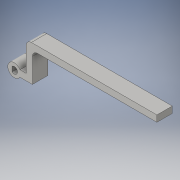
# Autodesk Inventor part: Rotator
Saved by Autodesk Inventor 2016 SP1 (Build 200210100, 210)
## iProperties
Created: 2016-04-06
Part Number: Rotator
Material: Generic
Document SubType Name: Modeling
Designer: jmehta38
Density: 1 g/cm^3
Appearance: Default
Author: jmehta38
Autodesk Inventor part; units mm, degrees
ref_plane "YZ Plane" through (0, 0, 0) normal (1, 0, 0) x (0, 1, 0)
ref_plane "XZ Plane" through (0, 0, 0) normal (0, 1, 0) x (-1, 0, 0)
ref_plane "XY Plane" through (0, 0, 0) normal (0, 0, 1) x (1, 0, 0)
sketch "Sketch2" plane through (0, 0, 0) normal (0, 0, 1) x (1, 0, 0)
  circle A0 centre (0, 0) radius 2
  circle A1 centre (0, 0) radius 4
  line L0 (3.4641, 2) -> (6.0041, 2)
  line L1 (6.0041, 2) -> (6.0041, -2.0132)
  line L2 (6.0041, -2.0132) -> (3.4564, -2.0132)
  line L3 (-1.3208, -1.5018) -> (-1.3208, 1.5018)
  dimension "d7" = 4
  dimension "d8" = 8
  dimension "d9" = 2.54
  dimension "d10" = 4.0132
  dimension "d11" = 2
  dimension "d25" = 1.3208
  constraints: 8 end point, 4 point on circle, 2 centre point, 2 coincident, 2 perpendicular, 1 horizontal, 1 vertical
  measures "d7" diameter of A0
  measures "d8" diameter of A1
  measures "d9" distance of L0.start L0.end
  measures "d10" distance of L0.end L1.end
  measures "d11" distance from line of L0 A0.centre
  measures "d25" distance from line of L3 point (0, 0)
extrude "Extrusion2" add sketch "Sketch2" along normal blind 9.398
sketch "Sketch3" plane through (6.0041, -2.0132, 0) normal (1, 0, 0) x (0, 0, -1)
  line L0 (-9.398, 0) -> (-9.398, 4.0132) projected
  line L1 (-9.398, 4.0132) -> (-9.398, 0)
  line L2 (-9.398, 0) -> (0, 0)
  line L3 (0, 0) -> (0, 4.0132) projected
  line L4 (0, 0) -> (0, 4.0132)
  line L5 (0, 4.0132) -> (-9.398, 4.0132) projected
  line L6 (0, 4.0132) -> (-9.398, 4.0132)
  point P0 (0, 2.0132)
  constraints: 8 end point, 3 perpendicular, 1 collinear
extrude "Extrusion3" add sketch "Sketch3" along normal blind 5.08
sketch "Sketch4" plane through (3.4641, 2, 9.398) normal (0, 1, 0) x (1, 0, 0)
  line L0 (0, 0) -> (7.62, 0) projected
  line L1 (7.62, 0) -> (3.81, 0)
  line L2 (3.81, 0) -> (3.81, 9.398)
  line L3 (3.81, 9.398) -> (7.62, 9.398)
  line L4 (7.62, 9.398) -> (7.62, 0)
  point P0 (-3.4641, 9.398)
  dimension "d16" = 3.81
  dimension "d17" = 9.398
  constraints: 8 end point, 3 perpendicular, 1 midpoint
  measures "d16" distance of L0.end L1.end
  measures "d17" distance between parallel lines of L3 L0
extrude "Extrusion4" add sketch "Sketch4" along normal blind 17.9303
sketch "Sketch5" plane through (11.0841, -2.0132, 0) normal (1, 0, 0) x (0, 0, -1)
  line L0 (0, 21.9435) -> (0, 18.04)
  line L1 (0, 18.04) -> (-9.398, 18.04)
  line L2 (-9.398, 18.04) -> (-9.398, 21.9435)
  line L3 (0, 0) -> (0, 21.9435) projected
  line L4 (-9.398, 21.9435) -> (0, 21.9435)
  point P0 (0, 2.0132)
  point P1 (-9.398, 21.9435)
  dimension "d29" = 9.398
  dimension "d30" = 3.9035
  dimension "d31" = 3.9035
  constraints: 8 end point, 2 perpendicular, 1 vertical
  measures "d29" distance of L0.end L1.end
  measures "d30" distance of L0.start L0.end
  measures "d31" distance of L2.end L1.end
extrude "Extrusion5" add sketch "Sketch5" along normal blind 76.2
fillet "Fillet1" radius 3.175 1 edges at (7.2741, 19.9303, 4.699)
fillet "Fillet2" radius 3.175 1 edges at (11.0841, 16.0268, 4.699)
sketch "Sketch6" plane through (0, 0, 9.398) normal (0, 0, 1) x (1, 0, 0)
  circle A0 centre (0, 0) radius 2 projected
  line L0 (-1.3208, -1.5018) -> (-1.3208, 1.5018)
  arc A1 (-1.3208, 1.5018) -> (-1.3208, -1.5018) centre (0, 0) ccw
  dimension "d26" = 1.3208
  constraints: 4 point on circle, 2 end point, 1 centre point, 1 concentric, 1 vertical
  measures "d26" distance from line of L0 point (0, 0)
extrude "Extrusion6" add sketch "Sketch6" against normal blind 9.398 contours L0 A0 picked at (-1.5423, 0.0807)
body "Solid2"
